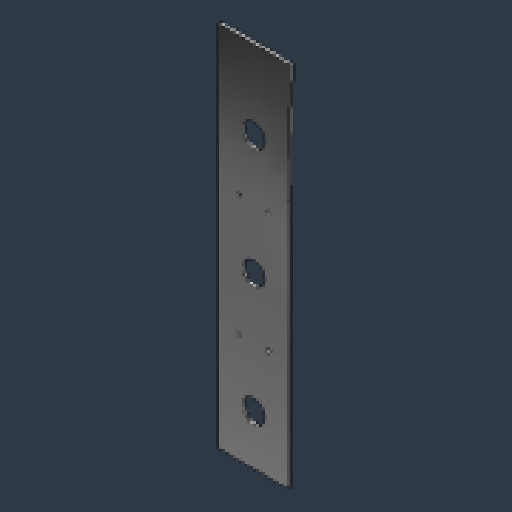
# Autodesk Inventor part: feeder_guide_plate
Saved by Autodesk Inventor 2024.3 (Build 283343000, 343)
## iProperties
Created: 2025-03-08
Part Number: feeder_guide_plate
Material: Aluminum 6061
Document SubType Name: Sheet Metal
Designer: marcu
Density: 2.7 g/cm^3
Sheet Metal Rule: Default
Appearance: Aluminum - Flat
Author: marcu
Autodesk Inventor part; units mm, degrees
ref_plane "YZ Plane" through (0, 0, 0) normal (1, 0, 0) x (0, 1, 0)
ref_plane "XZ Plane" through (0, 0, 0) normal (0, 1, 0) x (-1, 0, 0)
ref_plane "XY Plane" through (0, 0, 0) normal (0, 0, 1) x (1, 0, 0)
sketch "Sketch1" plane through (0, 0, 0) normal (0, 0, 1) x (1, 0, 0)
  line L0 (38.1, -158.75) -> (-38.1, -158.75)
  line L1 (-38.1, -158.75) -> (-38.1, 158.75)
  line L2 (-38.1, 158.75) -> (38.1, 158.75)
  line L3 (38.1, 158.75) -> (38.1, -158.75)
  line L4 (38.1, -158.75) -> (-38.1, 158.75) construction
  line L5 (-38.1, -158.75) -> (38.1, 158.75) construction
  line L6 (38.1, 158.75) -> (53.975, 311.15)
  line L7 (-38.1, 158.75) -> (-38.1, 311.15)
  line L8 (-38.1, 311.15) -> (53.975, 311.15)
  point P0 (0, 0)
  dimension "d0" = 76.2
  dimension "d1" = 317.5
  dimension "d2" = 92.075
  dimension "d3" = 152.4
  measures "d0" distance of L1.end L2.end
  measures "d1" distance of L0.end L1.end
  measures "d2" distance from line of L6.end L1
  measures "d3" distance from line of L2 L6.end
extrude "Plate1" add sketch "Sketch1" along normal blind 3.048
sketch "Sketch2" plane through (0, 0, 3.048) normal (0, 0, 1) x (1, 0, 0)
  line L0 (38.1, -158.75) -> (-38.1, -158.75) construction
  line L1 (-38.1, -158.75) -> (-38.1, 311.15) construction
  point P0 (0, 0)
  point P1 (6.35, -95.25)
  point P2 (0, -158.75)
  point P3 (6.35, 57.15)
  point P4 (6.35, 209.55)
  dimension "d5" = 63.5
  dimension "d8" = 152.4
  dimension "d29" = 44.45
  constraints: 1 midpoint, 1 vertical, 2 other
  measures "d5" distance from line of L0 point (6.35, -95.25)
  measures "d8" distance of point (6.35, -95.25) point (6.35, 57.15)
  measures "d29" distance from line of L1 point (6.35, -95.25)
hole "Hole1" at (6.35, -95.25, 3.048) at (6.35, 57.15, 3.048) at (6.35, 209.55, 3.048) direction (0, 0, -1) diameter 28.575 end through all
sketch "Sketch3" plane through (0, 0, 3.048) normal (0, 0, 1) x (1, 0, 0)
  circle A0 centre (6.35, 57.15) radius 14.2875 construction
  circle A1 centre (6.35, -95.25) radius 14.2875 construction
  line L0 (6.35, 57.15) -> (6.35, -95.25) construction
  line L1 (-12.7, -19.05) -> (25.4, -19.05) construction
  circle A2 centre (6.35, 209.55) radius 14.2875 construction
  line L2 (6.35, 57.15) -> (6.35, 209.55) construction
  line L3 (-12.7, 133.35) -> (25.4, 133.35) construction
  line L4 (6.35, 209.55) -> (6.35, 285.75) construction
  line L5 (-12.7, 285.75) -> (25.4, 285.75) construction
  point P0 (0, 0)
  point P1 (6.35, -19.05)
  point P2 (6.35, 133.35)
  dimension "d20" = 38.1
  dimension "d28" = 38.1
  dimension "d31" = 76.2
  dimension "d32" = 38.1
  constraints: 12 end point, 6 coincident, 5 midpoint, 3 horizontal, 3 vertical
  measures "d20" distance of L1.start L1.end
  measures "d28" distance of L3.start L3.end
  measures "d31" distance of L4.end L2.end
  measures "d32" distance of L5.start L5.end
hole "Hole2" at (-12.7, -19.05, 3.048) at (25.4, -19.05, 3.048) at (-12.7, 133.35, 3.048) at (25.4, 133.35, 3.048) at (-12.7, 285.75, 3.048) at (25.4, 285.75, 3.048) direction (0, 0, -1) diameter 5.1054 end through all clearance for "Flat Head Machine Screw (82)" size "#10" standard "Ansi Unified Screw Threads"
fillet "Corner Round1" radius 50.8 1 edges at (38.1, 158.75, 1.524)
equation "\"d18\" = Thickness"
equation "\"d28\" = d20"
equation "\"d4\" = Thickness"
equation "\"BendRadius\" = Thickness"
equation "\"BendReliefWidth\" = Thickness"
equation "\"BendReliefDepth\" = 0.5 * Thickness"
equation "\"CornerReliefSize\" = 4 * Thickness"
equation "\"MinimumRemnant\" = 2 * Thickness"
equation "\"TransitionRadius\" = BendRadius"
equation "\"JacobiRadiusSize\" = BendRadius"
equation "\"GapSize\" = Thickness"
equation "\"Thickness\" = 3.048"
body "Solid1"
